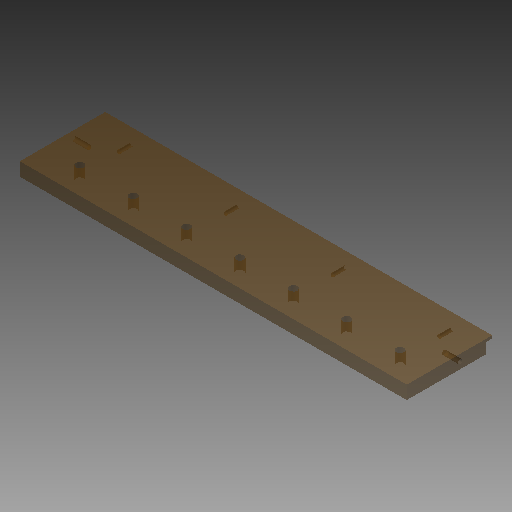
# Autodesk Inventor part: Tunnelwand
Saved by Autodesk Inventor 2018 (Build 220112000, 112)
## iProperties
Created: 2013-02-19
Part Number: Tunnelwand
Material: Polycarbonate, Clear
Document SubType Name: Modeling
Designer: Neef
Mass: 206.425 g
Surface Area: 450.436 cm^2
Volume: 172.021 cm^3
Density: 1.2 g/cm^3
Appearance: Polycarbonate - Smoked
Author: Neef
Autodesk Inventor part; units mm, degrees
ref_plane "YZ Plane" through (0, 0, 0) normal (1, 0, 0) x (0, 1, 0)
ref_plane "XZ Plane" through (0, 0, 0) normal (0, 1, 0) x (-1, 0, 0)
ref_plane "XY Plane" through (0, 0, 0) normal (0, 0, 1) x (1, 0, 0)
sketch "Skizze1" plane through (0, 0, 0) normal (0, 0, 1) x (1, 0, 0)
  line L0 (0, 44.8) -> (0, -44.8) projected
  line L1 (-203, 0) -> (203, 0) projected
  line L2 (-145, 32) -> (145, 32)
  line L3 (145, 32) -> (145, -32)
  line L4 (145, -32) -> (-145, -32)
  line L5 (-145, -32) -> (-145, 32)
  point P0 (0, 0)
  point P1 (0, 32)
  point P2 (-145, 0)
  dimension "d0" = 290
  dimension "d1" = 64
  constraints: 8 end point, 2 midpoint, 2 parallel, 2 point on line, 1 horizontal, 1 perpendicular
  measures "d0" distance of L2.start L2.end
  measures "d1" distance of L4.end L2.start
extrude "Extrusion1" add sketch "Skizze1" along normal blind 10
sketch "Skizze2" plane through (145, -32, 0) normal (1, 0, 0) x (0, 0, -1)
  line L0 (-10, 64) -> (-10, 0) projected
  line L1 (0, 0) -> (0, 64) projected
  line L2 (0, 64) -> (-10, 64) projected
  line L3 (0, 59) -> (-8, 59)
  line L4 (-8, 59) -> (-8, 64)
  point P0 (0, 32)
  dimension "d4" = 2
  dimension "d5" = 5
  constraints: 4 end point, 2 point on line, 1 parallel, 1 perpendicular
  measures "d4" distance between parallel lines of L0 L4
  measures "d5" distance of L3.end L4.end
extrude "Extrusion2" cut sketch "Skizze2" against normal through all
sketch "Skizze3" plane through (0, 0, 10) normal (0, 0, 1) x (1, 0, 0)
  line L0 (-145, -32) -> (-145, 32) projected
  line L1 (145, -32) -> (-145, -32) projected
  point P0 (0, 0)
  point P1 (-120, -12)
  dimension "d8" = 25
  dimension "d9" = 20
  measures "d8" distance from line of L0 point (-120, -12)
  measures "d9" distance from line of L1 point (-120, -12)
hole "Bohrung1" at (-120, -12, 10) direction (0, 0, -1) diameter 6 end through all
pattern_linear "Rechteckige Anordnung1" count 7 spacing 40 along (1, 0, 0) of "Bohrung1"
sketch "Skizze4" plane through (145, 27, 8) normal (0, 1, 0) x (1, 0, 0)
  line L0 (-290, 0) -> (-290, 8) projected
  line L1 (-290, 8) -> (0, 8) projected
  point P0 (-145, 8)
  point P1 (-265, 4)
  dimension "d20" = 25
  dimension "d21" = 4
  measures "d20" distance from line of L0 point (-265, 4)
  measures "d21" distance from line of L1 point (-265, 4)
hole "Bohrung2" at (-120, 27, 4) direction (0, -1, 0) diameter 2.459 depth 10 tip angle 118 thread size "M3x0.5" class "6H" standard "ISO Metric profile"
pattern_linear "Rechteckige Anordnung2" count 4 spacing 80 along (1, 0, 0) of "Bohrung2"
sketch "Skizze5" plane through (145, -32, 10) normal (1, 0, 0) x (0, 0, -1)
  line L0 (10, 0) -> (0, 0) projected
  point P0 (10, 32)
  point P1 (5, 40)
  dimension "d32" = 40
  measures "d32" distance from line of L0 point (5, 40)
hole "Bohrung3" at (145, 8, 5) direction (-1, 0, 0) diameter 3.242 depth 12 tip angle 118 thread size "M4x0.7" class "6H" standard "ISO Metric profile"
mirror "Spiegeln1" about plane through (0, 0, 0) normal (1, 0, 0) of "Bohrung3"
